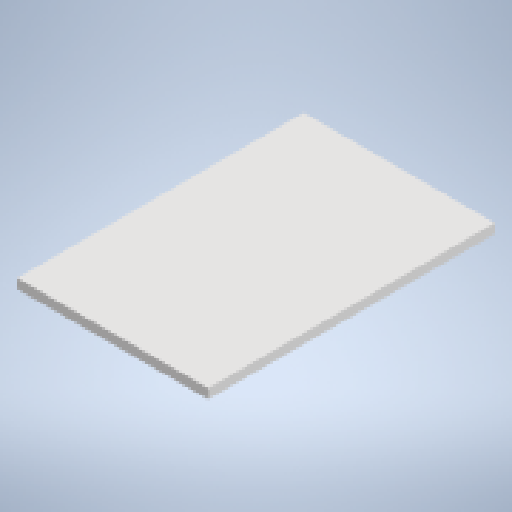
# Autodesk Inventor part: FlexBlockWheelSupport
Saved by Autodesk Inventor 2023 (Build 270158000, 158)
## iProperties
Created: 2023-03-20
Part Number: FlexBlockWheelSupport
Material: Generic
Document SubType Name: Modeling
Designer: Nathann
Density: 1 g/cm^3
Appearance: Default
Author: Nathann
Autodesk Inventor part; units mm, degrees
ref_plane "YZ Plane" through (0, 0, 0) normal (1, 0, 0) x (0, 1, 0)
ref_plane "XZ Plane" through (0, 0, 0) normal (0, 1, 0) x (-1, 0, 0)
ref_plane "XY Plane" through (0, 0, 0) normal (0, 0, 1) x (1, 0, 0)
sketch "Sketch1" plane through (0, 0, 0) normal (0, 1, 0) x (-1, 0, 0)
  line L0 (0, 0) -> (-100, 0)
  line L1 (-100, 0) -> (-100, -150)
  line L2 (-100, -150) -> (0, -150)
  line L3 (0, -150) -> (0, 0)
  dimension "d0" = 150
  dimension "d1" = 100
  constraints: 8 end point, 2 parallel, 1 horizontal, 1 perpendicular
  measures "d0" distance of L0.end L1.end
  measures "d1" distance of L0.start L0.end
extrude "Extrusion1" add sketch "Sketch1" along normal blind 5
sketch "Sketch2" plane through (0, 5, 0) normal (0, 1, 0) x (1, 0, 0)
  circle A0 centre (65.8462, 111.6036) radius 1.5 projected
  circle A1 centre (61.6036, 115.8462) radius 1.5 projected
  circle A2 centre (38.3964, 115.8462) radius 1.5 projected
  circle A3 centre (34.1538, 111.6036) radius 1.5 projected
  circle A4 centre (34.1538, 88.3964) radius 1.5 projected
  circle A5 centre (38.3964, 84.1538) radius 1.5 projected
  circle A6 centre (61.6036, 84.1538) radius 1.5 projected
  circle A7 centre (65.8462, 88.3964) radius 1.5 projected
  point P0 (0, 0)
extrude "Extrusion2" cut sketch "Sketch2" against normal blind 5
sketch "Sketch3" plane through (0, 5, 0) normal (0, 1, 0) x (1, 0, 0)
  circle A0 centre (5, 145) radius 1.5 projected
  circle A1 centre (5, 5) radius 1.5 projected
  circle A2 centre (95, 5) radius 1.5 projected
  point P0 (0, 0)
extrude "Extrusion3" cut sketch "Sketch3" against normal blind 5
equation "\"d2\" = woodThickness"
equation "\"d4\" = woodThickness"
equation "\"d6\" = woodThickness"
equation "\"bladeLenghtFlexRatio\" = 0.05"
equation "\"bladeThickness\" = 1"
equation "\"woodThickness\" = 5"
equation "\"colRadius\" = 3"
equation "\"M3Hole\" = 3"
body "Solid1"
